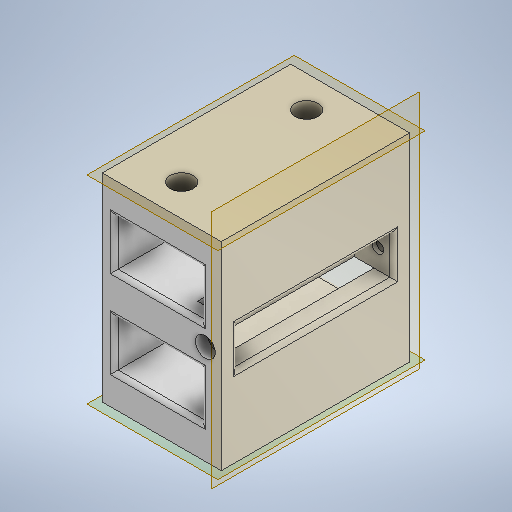
# Autodesk Inventor part: motor_rot_born1
Saved by Autodesk Inventor 2025.2 (Build 292293000, 293)
## iProperties
Created: 2024-12-22
Part Number: motor_rot_born1
Material: 一般
Document SubType Name: Modeling
Designer: mahhy
Density: 1 g/cm^3
Appearance: 既定
Author: mahhy
## iProperties of the stored document motor_rot_born1_3D プリント.ipt
Created: 2024-12-22
Part Number: motor_rot_born1_3D プリント
Material: 一般
Document SubType Name: Modeling
Designer: mahhy
Density: 1 g/cm^3
Appearance: 既定
Author: mahhy
Autodesk Inventor part; units mm, degrees
ref_plane "YZ Plane" through (0, 0, 0) normal (1, 0, 0) x (0, 1, 0)
ref_plane "XZ Plane" through (0, 0, 0) normal (0, 1, 0) x (-1, 0, 0)
ref_plane "XY Plane" through (0, 0, 0) normal (0, 0, 1) x (1, 0, 0)
sketch "スケッチ1" plane through (0, 0, 0) normal (0, 1, 0) x (-1, 0, 0)
  line L0 (0, 0) -> (-30, 0)
  line L1 (-30, 0) -> (-30, -47.5)
  line L2 (-30, -47.5) -> (0, -47.5)
  line L3 (0, -47.5) -> (0, 0)
  dimension "d0" = 30
  dimension "d1" = 47.5
  constraints: 8 end point, 2 parallel, 1 horizontal, 1 perpendicular
  measures "d0" distance of L2.end L1.end
  measures "d1" distance of L1.end L0.end
extrude "押し出し1" add sketch "スケッチ1" along normal blind 50
ref_plane "作業平面1" through (30, 0, 0) normal (1, 0, 0) x (0, 0, -1)
sketch "スケッチ2" plane through (30, 0, 0) normal (1, 0, 0) x (0, 0, -1)
  line L0 (4, 30) -> (43.5, 30)
  line L1 (43.5, 30) -> (43.5, 20)
  line L2 (43.5, 20) -> (4, 20)
  line L3 (4, 20) -> (4, 30)
  line L4 (0, 0) -> (0, 50) projected
  line L5 (0, 0) -> (0, 50) projected
  line L6 (0, 50) -> (47.5, 50) projected
  point P0 (0, 25)
  point P1 (4, 25)
  point P2 (0, 25)
  point P3 (23.75, 30)
  point P4 (23.75, 50)
  point P5 (23.75, 50)
  dimension "d5" = 39.5
  dimension "d6" = 10
  dimension "d7" = 0
  dimension "d8" = 0
  constraints: 8 end point, 6 midpoint, 2 parallel, 1 horizontal, 1 perpendicular
  measures "d5" distance of L1.end L2.end
  measures "d6" distance of L0.end L1.end
  measures "d7" vertical distance of point (0, 25) point (4, 25)
  measures "d8" horizontal distance of point (23.75, 30) point (23.75, 50)
extrude "押し出し2" cut sketch "スケッチ2" against normal blind 10
sketch "スケッチ3" plane through (0, 0, 0) normal (0, 0, 1) x (1, 0, 0)
  line L0 (3, 42) -> (25, 42)
  line L1 (25, 42) -> (25, 30)
  line L2 (25, 30) -> (3, 30)
  line L3 (3, 30) -> (3, 42)
  line L4 (0, 50) -> (30, 50) projected
  line L5 (3, 20) -> (25, 20)
  line L6 (25, 20) -> (25, 8)
  line L7 (25, 8) -> (3, 8)
  line L8 (3, 8) -> (3, 20)
  line L9 (0, 0) -> (30, 0) projected
  line L10 (0, 0) -> (0, 50) projected
  point P0 (14, 42)
  point P1 (15, 50)
  point P2 (15, 50)
  point P3 (14, 8)
  point P4 (15, 0)
  point P5 (15, 0)
  dimension "d11" = 22
  dimension "d12" = 12
  dimension "d13" = 8
  dimension "d14" = 22
  dimension "d15" = 12
  dimension "d16" = 8
  dimension "d48" = 3
  dimension "d49" = 3
  constraints: 16 end point, 6 midpoint, 4 parallel, 2 horizontal, 2 perpendicular
  measures "d11" distance of L1.end L2.end
  measures "d12" distance of L0.end L1.end
  measures "d13" distance between parallel lines of L4 L0
  measures "d14" distance of L6.end L7.end
  measures "d15" distance of L5.end L6.end
  measures "d16" distance between parallel lines of L9 L7
  measures "d48" distance between parallel lines of L10 L3
  measures "d49" distance between parallel lines of L10 L8
extrude "押し出し3" cut sketch "スケッチ3" against normal through all
ref_plane "作業平面2" through (0, 50, 0) normal (0, 1, 0) x (1, 0, 0)
sketch "スケッチ4" plane through (0, 50, 0) normal (0, 1, 0) x (1, 0, 0)
  line L0 (30, 57) -> (30, -9.5) projected
  line L1 (30, 47.5) -> (0, 47.5) projected
  line L2 (0, 0) -> (30, 0) projected
  line L3 (0, 47.5) -> (0, 0) projected
  point P0 (12, 39.5)
  point P1 (12, 8)
  dimension "d24" = 8
  dimension "d25" = 8
  dimension "d52" = 12
  dimension "d53" = 12
  measures "d24" distance from line of L1 point (12, 39.5)
  measures "d25" distance from line of L2 point (12, 8)
  measures "d52" distance from line of L3 point (12, 39.5)
  measures "d53" distance from line of L3 point (12, 8)
hole "穴1" at (12, 50, -39.5) at (12, 50, -8) direction (0, -1, 0) diameter 5.8 depth 7
sketch "スケッチ5" plane through (0, 0, 0) normal (0, 0, 1) x (1, 0, 0)
  line L0 (30, 0) -> (30, 50) projected
  circle A0 centre (26, 25) radius 1.5
  point P0 (0, 0)
  point P1 (30, 25)
  point P2 (30, 25)
  dimension "d33" = 4
  dimension "d34" = 3
  constraints: 2 coincident, 1 centre point, 1 midpoint
  measures "d33" distance of point (30, 25) point (26, 25)
  measures "d34" diameter of A0
hole "穴2" at (26, 25, 0) direction (0, 0, -1) diameter 2.85 end through all
sketch "スケッチ6" plane through (0, 0, 0) normal (0, 0, 1) x (1, 0, 0)
  circle A0 centre (26, 25) radius 1.425 projected
  circle A1 centre (26, 25) radius 2.5
  point P0 (0, 0)
  dimension "d42" = 5
  constraints: 2 coincident, 1 centre point
  measures "d42" diameter of A1
extrude "押し出し4" cut sketch "スケッチ6" against normal blind 3 contours A0 | A1
sketch "スケッチ7" plane through (30, 0, -47.5) normal (0, 0, -1) x (-1, 0, 0)
  circle A0 centre (4, 25) radius 1.425 projected
  circle A1 centre (4, 25) radius 2.5
  point P0 (30, 0)
  dimension "d45" = 5
  constraints: 1 centre point, 1 coincident
  measures "d45" diameter of A1
extrude "押し出し5" cut sketch "スケッチ7" against normal blind 3 contours A0 | A1
fillet "フィレット1" radius 1 4 edges at (30, 25, -43.5) (30, 30, -23.75) (30, 20, -23.75) (30, 25, -4)
fillet "フィレット2" radius 1 16 edges at (3, 36, 0) (14, 42, 0) (14, 30, 0) (25, 36, 0) (25, 14, 0) (14, 20, 0) (3, 14, 0) (14, 8, 0) (3, 36, -47.5) (14, 42, -47.5) (25, 36, -47.5) (14, 30, -47.5) (14, 20, -47.5) (3, 14, -47.5) (25, 14, -47.5) (14, 8, -47.5)
ref_plane "作業平面3" through (0, 0, 0) normal (0, -1, 0) x (1, 0, 0)
sketch "スケッチ8" plane through (0, 0, 0) normal (0, -1, 0) x (1, 0, 0)
  circle A0 centre (12, -8) radius 2.9 projected
  circle A1 centre (12, -39.5) radius 2.9 projected
  point P0 (0, 0)
  constraints: 2 coincident
hole "穴3" at (12, 0, -8) at (12, 0, -39.5) direction (0, 1, 0) diameter 5.8 depth 7
